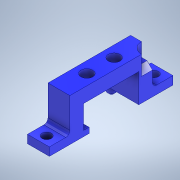
# Autodesk Inventor part: Servo mount Right
Saved by Autodesk Inventor 2022.6 (Build 266554000, 554)
## iProperties
Created: 2024-11-05
Part Number: Servo mount Right
Material: Generic
Document SubType Name: Modeling
Designer: Admin
Density: 1 g/cm^3
Appearance: Blue - Wall Paint - Glossy
Author: Admin
Autodesk Inventor part; units mm, degrees
ref_plane "YZ Plane" through (0, 0, 0) normal (1, 0, 0) x (0, 1, 0)
ref_plane "XZ Plane" through (0, 0, 0) normal (0, 1, 0) x (-1, 0, 0)
ref_plane "XY Plane" through (0, 0, 0) normal (0, 0, 1) x (1, 0, 0)
sketch "Sketch1" plane through (0, 0, 0) normal (1, 0, 0) x (0, 1, 0)
  line L0 (0, 0) -> (15.5, 0)
  line L1 (15.5, 0) -> (15.5, -5)
  line L2 (15.5, -5) -> (0, -5)
  line L3 (0, -5) -> (0, 0)
  line L4 (15.5, 0) -> (10.5, 0)
  line L5 (10.5, 0) -> (10.5, 20.2)
  line L6 (10.5, 20.2) -> (15.5, 20.2)
  line L7 (15.5, 20.2) -> (15.5, 0)
  line L8 (15.5, 20.2) -> (0, 20.2)
  line L9 (0, 20.2) -> (0, 25.2)
  line L10 (0, 25.2) -> (15.5, 25.2)
  line L11 (15.5, 25.2) -> (15.5, 20.2)
  line L12 (2, 20.2) -> (0, 20.2)
  line L13 (0, 20.2) -> (0, 18.2)
  line L14 (0, 18.2) -> (2, 18.2)
  line L15 (2, 18.2) -> (2, 20.2)
  line L16 (0, 0) -> (2, 0)
  line L17 (2, 0) -> (2, 2)
  line L18 (2, 2) -> (0, 2)
  line L19 (0, 2) -> (0, 0)
  dimension "d0" = 5
  dimension "d2" = 5
  dimension "d3" = 20.2
  dimension "d4" = 5
  dimension "d16" = 10.5
  dimension "d23" = 2
  dimension "d24" = 2
  dimension "d59" = 2
  dimension "d60" = 2
  constraints: 40 end point, 11 parallel, 5 perpendicular, 4 horizontal, 2 point on line
  measures "d0" distance of L0.end L1.end
  measures "d2" distance of L5.end L6.end
  measures "d3" distance of L6.end L0.end
  measures "d4" distance of L8.end L9.end
  measures "d16" distance between parallel lines of L3 L5
  measures "d23" distance of L14.end L13.end
  measures "d24" distance of L14.end L12.start
  measures "d59" distance of L0.start L16.end
  measures "d60" distance of L17.end L16.end
extrude "Extrusion1" add sketch "Sketch1" along normal blind 8 contours L0 L1 L2 L3 | L5 L6 L7 L0 | L8 L9 L10 L11 L6 | L15 L14 L13 L8
sketch "Sketch2" plane through (0, 15.5, 25.2) normal (0, 1, 0) x (1, 0, 0)
  line L0 (0, 0) -> (8, 0) construction
  line L1 (4.1, 0) -> (4.1, 30.2) construction
  line L2 (0, 30.2) -> (8, 30.2) construction
  line L3 (0, 30.2) -> (0, 0) construction
  line L4 (0, 30.2) -> (0, 0) construction
  line L5 (0, 0) -> (8, 0) construction
  line L6 (8, 30.2) -> (8, 0) construction
  line L7 (0, 30.2) -> (8, 30.2) construction
  line L8 (4.1, 15.1) -> (1.5202, 15.1)
  point P0 (0, 25.2)
  point P1 (4.1, 10.1)
  point P2 (4.1, 20.1)
  dimension "d8" = 10
  dimension "d64" = 3.9
  constraints: 4 end point, 4 point on line, 1 horizontal, 1 midpoint, 1 symmetric about line, 1 vertical
  measures "d8" distance of point (4.1, 10.1) point (4.1, 20.1)
  measures "d64" distance between parallel lines of L6 L1
hole "Hole1" at (4.1, 15.5, 15.1) at (4.1, 15.5, 5.1) direction (0, -1, 0) diameter 4.3 depth 10 tip angle 118
sketch "Sketch6" plane through (0, 0, -5) normal (0, -1, 0) x (1, 0, 0)
  line L0 (0, 5) -> (0, 0) projected
  line L1 (0, 0) -> (8, 0) projected
  line L2 (8, 5) -> (8, 0) projected
  line L3 (0, 5) -> (8, 5) projected
  line L4 (8, 0) -> (0, 0)
  line L5 (0, 0) -> (0, -7.5)
  line L6 (0, -7.5) -> (8, -7.5)
  line L7 (8, -7.5) -> (8, 0)
  line L8 (0, 5) -> (8, 5) projected
  line L9 (0, 0) -> (0, 30.2) projected
  line L10 (0, 5) -> (0, 0)
  line L11 (0, 0) -> (-7.5, 0)
  line L12 (-7.5, 0) -> (-7.5, 5)
  line L13 (-7.5, 5) -> (0, 5)
  line L14 (0, 30.2) -> (0, 23.2) projected
  line L15 (0, 23.2) -> (8, 23.2) projected
  line L16 (8, 30.2) -> (8, 23.2) projected
  line L17 (0, 30.2) -> (8, 30.2) projected
  line L18 (0, 30.2) -> (8, 30.2) projected
  line L19 (8, 30.2) -> (0, 30.2)
  line L20 (0, 30.2) -> (0, 37.7)
  line L21 (0, 37.7) -> (8, 37.7)
  line L22 (8, 37.7) -> (8, 30.2)
  line L23 (0, 30.2) -> (0, 23.2) projected
  line L24 (0, 23.2) -> (8, 23.2) projected
  line L25 (0, 30.2) -> (0, 23.2)
  line L26 (0, 23.2) -> (-7.5, 23.2)
  line L27 (-7.5, 23.2) -> (-7.5, 30.2)
  line L28 (-7.5, 30.2) -> (0, 30.2)
  point P0 (0, 26.8752)
  dimension "d31" = 7.5
  dimension "d35" = 7.5
  dimension "d61" = 7.5
  dimension "d62" = 7.5
  constraints: 32 end point, 8 parallel, 5 perpendicular, 2 collinear, 1 horizontal
  measures "d31" distance of L0.end L5.end
  measures "d35" distance of L0.end L11.end
  measures "d61" distance of L9.end L20.end
  measures "d62" distance of L14.end L26.end
extrude "Extrusion4" add sketch "Sketch6" against normal blind 3 contours L0 L11 L12 L13 | L1 L7 L6 L5 | L20 L21 L22 L17
fillet "Fillet1" radius 1.5 4 edges at (0, 1.5, -5) (0, 3, -2.5) (4, 3, -5) (4, 3, 25.2)
sketch "Sketch8" plane through (0, 0, -12.5) normal (0, -1, 0) x (1, 0, 0)
  line L0 (0, 6) -> (0, 0) projected
  line L1 (0, 0) -> (8, 0) projected
  line L2 (8, 12.5) -> (8, 0) projected
  line L3 (-7.5, 12.5) -> (8, 12.5) projected
  line L4 (-7.5, 12.5) -> (-7.5, 7.5) projected
  line L5 (-7.5, 7.5) -> (-1.5, 7.5) projected
  arc A0 (0, 6) -> (-1.5, 7.5) centre (-1.5, 6) ccw projected
  line L6 (8, 0) -> (0, 0) construction
  line L7 (4, 0) -> (4, 12.5) construction
  line L8 (0, 12.5) -> (8, 12.5) construction
  line L9 (-7.5, 12.5) -> (-7.5, 7.5) construction
  line L10 (-7.5, 10) -> (8, 10) construction
  line L11 (8, 7.5) -> (8, 37.7) construction
  line L12 (0, 30.7) -> (8, 30.7) projected
  line L13 (8, 30.7) -> (8, 45.2) projected
  line L14 (8, 45.2) -> (0, 45.2) projected
  line L15 (0, 45.2) -> (0, 30.7) projected
  circle A1 centre (-4.5, 10) radius 1.45
  point P0 (4, 3)
  point P1 (4, 42.2)
  dimension "d49" = 3
  dimension "d58" = 12.5
  dimension "d63" = 3
  dimension "d71" = 2.9
  constraints: 4 end point, 3 midpoint, 3 point on line, 1 centre point, 1 coincident, 1 perpendicular, 1 vertical alignment
  measures "d49" distance from line of L6 point (4, 3)
  measures "d58" distance from line of L2 point (-4.5, 10)
  measures "d63" distance from line of L14 point (4, 42.2)
  measures "d71" diameter of A1
hole "Hole3" at (4, 0, -9.5) at (4, 0, 29.7) direction (0, 1, 0) diameter 3.4 depth 10 tip angle 118
sketch "Sketch9" plane through (0, 15.5, 25.2) normal (0, 1, 0) x (1, 0, 0)
  circle A0 centre (4.1, 10.1) radius 2.15 projected
  circle A1 centre (4.1, 20.1) radius 2.15 projected
  line L0 (0, 30.2) -> (0, 0) projected
  line L1 (0, 0) -> (8, 0) projected
  line L2 (8, 30.2) -> (8, 0) projected
  line L3 (0, 30.2) -> (8, 30.2) projected
  line L4 (0, 30.2) -> (8, 30.2) projected
  circle A2 centre (8, 30.2) radius 4
  point P0 (0, 25.2)
  dimension "d65" = 8
  constraints: 1 centre point, 1 coincident
  measures "d65" diameter of A2
extrude "Extrusion5" cut sketch "Sketch9" against normal blind 5 contours A2 L2 L3 | L3 L2 A2
chamfer "Chamfer1" distance 2 angle 45 1 edges at (8, 10.5, -3)
extrude "Extrusion6" add sketch "Sketch8" along normal blind 3.8 contours A1
chamfer "Chamfer2" distance 0.8 angle 45 1 edges at (-5.95, -3.8, -2.5)
body "Solid1"
